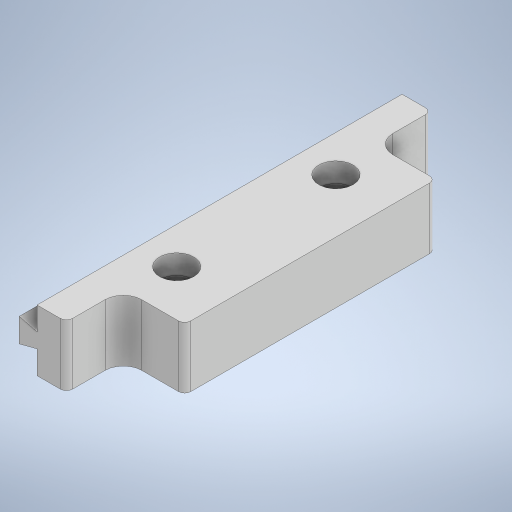
# Autodesk Inventor part: tyl
Saved by Autodesk Inventor 2023 (Build 270158000, 158)
## iProperties
Created: 2024-04-25
Part Number: tyl
Material: Ogólny
Document SubType Name: Modeling
Designer: Kamil
Density: 1 g/cm^3
Appearance: Domyślna
Author: Kamil
Autodesk Inventor part; units mm, degrees
ref_plane "YZ Plane" through (0, 0, 0) normal (1, 0, 0) x (0, 1, 0)
ref_plane "XZ Plane" through (0, 0, 0) normal (0, 1, 0) x (-1, 0, 0)
ref_plane "XY Plane" through (0, 0, 0) normal (0, 0, 1) x (1, 0, 0)
sketch "Szkic1" plane through (0, 0, 0) normal (0, 1, 0) x (-1, 0, 0)
  line L0 (-1, -9) -> (-6, -9)
  line L1 (-6, -9) -> (-6, -69)
  line L2 (-6, -69) -> (-1, -69)
  line L3 (-1, -69) -> (-1, -9)
  point P0 (0, 0)
  dimension "d0" = 5
  dimension "d1" = 60
  constraints: 8 end point, 2 parallel, 1 horizontal, 1 perpendicular
  measures "d0" distance of L2.end L1.end
  measures "d1" distance of L1.end L0.end
extrude "Wyciągnięcie proste1" add sketch "Szkic1" along normal blind 10
sketch "Szkic2" plane through (1, 0, -9) normal (0, 0, 1) x (1, 0, 0)
  line L0 (0, 0) -> (5, 0) projected
  line L1 (5, 0) -> (5, 10) projected
  line L2 (0, 10) -> (5, 10) projected
  line L3 (0, 0) -> (0, 10) projected
  line L4 (-2.9, 6.95) -> (-2.9, 3.05)
  line L5 (0, 6.2) -> (0, 3.8)
  line L6 (-2.9, 6.95) -> (0, 6.2)
  line L7 (0, 3.8) -> (-2.9, 3.05)
  point P0 (-1, 0)
  point P1 (-2.9, 5)
  point P2 (0, 5)
  point P3 (0, 5)
  point P4 (0, 5)
  dimension "d7" = 3.9
  dimension "d8" = 2.4
  dimension "d9" = 2.9
  constraints: 8 end point, 3 midpoint, 2 coincident, 1 horizontal alignment, 1 parallel, 1 vertical, 1 vertical alignment
  measures "d7" distance of L4.start L4.end
  measures "d8" distance of L5.start L5.end
  measures "d9" distance between parallel lines of L4 L5
extrude "Wyciągnięcie proste2" add sketch "Szkic2" against normal up to surface (60 mm away) contours L7 L4 L6 L3
sketch "Szkic3" plane through (0, 10, 0) normal (0, 1, 0) x (1, 0, 0)
  line L0 (16, 18.3) -> (6, 18.3)
  line L1 (6, 18.3) -> (6, 59.7)
  line L2 (6, 59.7) -> (16, 59.7)
  line L3 (16, 59.7) -> (16, 18.3)
  line L4 (6, 9) -> (6, 69) projected
  point P0 (0, 0)
  point P1 (6, 39)
  point P2 (6, 39)
  point P3 (6, 39)
  dimension "d12" = 41.4
  dimension "d13" = 10
  constraints: 8 end point, 3 midpoint, 2 coincident, 2 parallel, 1 horizontal, 1 perpendicular
  measures "d12" distance of L0.end L1.end
  measures "d13" distance between parallel lines of L1 L3
extrude "Wyciągnięcie proste3" add sketch "Szkic3" against normal blind 10
sketch "Szkic4" plane through (0, 10, 0) normal (0, 1, 0) x (1, 0, 0)
  line L0 (6, 9) -> (6, 18.3) projected
  line L1 (6, 18.3) -> (16, 18.3) projected
  line L2 (16, 18.3) -> (16, 59.7) projected
  line L3 (16, 59.7) -> (6, 59.7) projected
  line L4 (6, 59.7) -> (6, 69) projected
  line L5 (6, 69) -> (1, 69) projected
  line L6 (1, 69) -> (1, 9) projected
  line L7 (1, 9) -> (6, 9) projected
  line L8 (7, 26) -> (7, 52)
  point P0 (0, 0)
  point P1 (7, 39)
  point P2 (1, 39)
  dimension "d16" = 6
  dimension "d17" = 6
  dimension "d18" = 26
  constraints: 2 end point, 2 midpoint, 1 horizontal alignment
  measures "d16" distance from line of L6 L8.start
  measures "d17" distance from line of L6 L8.end
  measures "d18" distance of L8.end L8.start
hole "Otwór1" at (7, 10, -26) at (7, 10, -52) direction (0, -1, 0) diameter 3.2 end through all counterbore diameter 5.6 counterbore depth 3.2
sketch "Szkic5" plane through (0, 10, 0) normal (0, 1, 0) x (1, 0, 0)
  line L0 (1, 69) -> (-1.9, 69) projected
  line L1 (6, 69) -> (1, 69) projected
  line L2 (16, 59.7) -> (6, 59.7) projected
  line L3 (6, 59.7) -> (6, 69) projected
  line L4 (16, 18.3) -> (16, 59.7) projected
  line L5 (6, 18.3) -> (16, 18.3) projected
  line L6 (1, 9) -> (6, 9) projected
  line L7 (1, 9) -> (-1.9, 9) projected
  line L8 (6, 9) -> (6, 18.3) projected
  line L9 (-1.9, 68.8) -> (1, 68.8)
  line L10 (1, 68.8) -> (5.8, 68.8)
  line L11 (5.8, 68.8) -> (5.8, 59.5)
  line L12 (5.8, 59.5) -> (15.8, 59.5)
  line L13 (15.8, 59.5) -> (15.8, 18.5)
  line L14 (15.8, 18.5) -> (5.8, 18.5)
  line L15 (5.8, 18.5) -> (5.8, 9.2)
  line L16 (5.8, 9.2) -> (1, 9.2)
  line L17 (1, 9.2) -> (-1.9, 9.2)
  line L18 (-1.9, 9) -> (-1.9, 9.2)
  line L19 (-1.9, 68.8) -> (-1.9, 69)
  point P0 (0, 0)
  dimension "d26" = 0.2
  constraints: 22 end point, 1 collinear, 1 perpendicular, 8 other
  measures "d26" distance between parallel lines of L3 L11
extrude "Wyciągnięcie proste4" cut sketch "Szkic5" against normal through all
fillet "Zaokrąglenie1" radius 3 2 edges at (5.8, 5, -18.5) (5.8, 5, -59.5)
fillet "Zaokrąglenie2" radius 1 4 edges at (5.8, 5, -9.2) (15.8, 5, -18.5) (15.8, 5, -59.5) (5.8, 5, -68.8)
